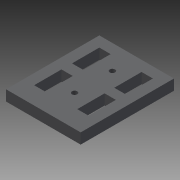
# Autodesk Inventor part: spoolHolderHolder
Saved by Autodesk Inventor 2013 (Build 170138000, 138)
## iProperties
Created: 2015-01-14
Part Number: spoolHolderHolder
Material: Generic
Document SubType Name: Modeling
Designer: dzban
Density: 1 g/cm^3
Author: dzban
Autodesk Inventor part; units mm, degrees
ref_plane "YZ Plane" through (0, 0, 0) normal (1, 0, 0) x (0, 1, 0)
ref_plane "XZ Plane" through (0, 0, 0) normal (0, 1, 0) x (-1, 0, 0)
ref_plane "XY Plane" through (0, 0, 0) normal (0, 0, 1) x (1, 0, 0)
sketch "Sketch1" plane through (0, 0, 0) normal (0, 0, 1) x (1, 0, 0)
  line L0 (-9.2194, -2.0534) -> (-9.2194, -17.5534)
  line L1 (-9.2194, -17.5534) -> (-15.6194, -17.5534)
  line L2 (-15.6194, -17.5534) -> (-15.6194, -2.0534)
  line L3 (-15.6194, -2.0534) -> (-9.2194, -2.0534)
  line L4 (-9.2194, 19.4466) -> (-9.2194, 3.9466)
  line L5 (-9.2194, 3.9466) -> (-15.6194, 3.9466)
  line L6 (-15.6194, 3.9466) -> (-15.6194, 19.4466)
  line L7 (-15.6194, 19.4466) -> (-9.2194, 19.4466)
  line L8 (14.7806, 19.4466) -> (14.7806, 3.9466)
  line L9 (14.7806, 3.9466) -> (8.3806, 3.9466)
  line L10 (8.3806, 3.9466) -> (8.3806, 19.4466)
  line L11 (8.3806, 19.4466) -> (14.7806, 19.4466)
  line L12 (14.7806, -1.568) -> (14.7806, -17.068)
  line L13 (14.7806, -17.068) -> (8.3806, -17.068)
  line L14 (8.3806, -17.068) -> (8.3806, -1.568)
  line L15 (8.3806, -1.568) -> (14.7806, -1.568)
  line L16 (20.7806, -27.5534) -> (20.7806, 25.4466)
  line L17 (20.7806, 25.4466) -> (-21.6194, 25.4466)
  line L18 (-21.6194, 25.4466) -> (-21.6194, -27.5534)
  line L19 (-21.6194, -27.5534) -> (20.7806, -27.5534)
  circle A0 centre (-0.4194, 11.6966) radius 1.5
  circle A1 centre (-0.4194, -9.8034) radius 1.5
  point P0 (0, 0)
  constraints: 40 end point, 2 centre point
extrude "Extrusion1" add sketch "Sketch1" along normal blind 6
body "Solid1"
